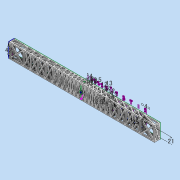
# Autodesk Inventor part: hashi1shado
Saved by Autodesk Inventor 2022 (Build 260153000, 153)
## iProperties
Created: 2024-05-14
Part Number: hashi1shado
Material: 一般
Document SubType Name: Modeling
Designer: ktamu
Density: 1 g/cm^3
Appearance: 既定
Mass: 151.289 g
Surface Area: 1319.93 cm^2
Volume: 151.289 cm^3
Author: ktamu
Autodesk Inventor part; units mm, degrees
ref_plane "YZ Plane" through (0, 0, 0) normal (1, 0, 0) x (0, 1, 0)
ref_plane "XZ Plane" through (0, 0, 0) normal (0, 1, 0) x (-1, 0, 0)
ref_plane "XY Plane" through (0, 0, 0) normal (0, 0, 1) x (1, 0, 0)
sketch "スケッチ2" plane through (0, 0, 0) normal (1, 0, 0) x (0, 1, 0)
  line L0 (25, 10) -> (-25, 10)
  line L1 (-25, 10) -> (-25, -10)
  line L2 (-25, -10) -> (25, -10)
  line L3 (25, -10) -> (25, 10)
  line L4 (25, 10) -> (-25, -10) construction
  line L5 (-25, 10) -> (25, -10) construction
  point P0 (0, 0)
  dimension "d4" = 50
  dimension "d5" = 20
  constraints: 12 end point, 2 midpoint, 2 parallel, 1 horizontal, 1 perpendicular
  measures "d4" distance of L2.end L1.end
  measures "d5" distance of L1.end L0.end
extrude "押し出し2" add sketch "スケッチ2" along normal mid plane 500
sketch "スケッチ3" plane through (-250, -25, 10) normal (0, 0, 1) x (1, 0, 0)
  circle A0 centre (250, 25) radius 5
  dimension "d8" = 10
  constraints: 1 centre point, 1 coincident
  measures "d8" diameter of A0
extrude "押し出し3" add sketch "スケッチ3" along normal blind 2
sketch "SCLeft" plane through (-250, 0, 0) normal (-1, 0, 0) x (0, 0, 1)
  line L0 (10, 25) -> (10, -25) projected
  line L1 (-10, 25) -> (10, 25)
  line L2 (10, 25) -> (10, -25)
  line L3 (10, -25) -> (-10, -25)
  line L4 (-10, -25) -> (-10, 25)
  line L5 (-10, 25) -> (10, -25) construction
  line L6 (10, 25) -> (-10, -25) construction
  line L7 (-6, 21) -> (6, 21)
  line L8 (6, 21) -> (6, -21)
  line L9 (6, -21) -> (-6, -21)
  line L10 (-6, -21) -> (-6, 21)
  line L11 (-6, 21) -> (-1.04, 3.6401) construction
  line L12 (6, 21) -> (-6, -21) construction
  line L13 (7.4154, 0) -> (4.3427, 0)
  line L14 (2.08, 0) -> (6, -13.7199)
  line L15 (-3.92, 21) -> (0, 7.2801)
  line L16 (-6, 21) -> (-1.04, 3.6401)
  line L17 (1.04, -3.6401) -> (6, -21)
  line L18 (-6, 13.7199) -> (-2.08, 0)
  line L19 (0, -7.2801) -> (3.92, -21)
  line L20 (0, 7.2801) -> (3.92, 21)
  line L21 (-6, -13.7199) -> (-2.08, 0)
  line L22 (-3.92, -21) -> (0, -7.2801)
  line L23 (2.08, 0) -> (6, 13.7199)
  point P0 (0, 0)
  dimension "d47" = 12
  dimension "d48" = 42
  constraints: 46 end point, 8 parallel, 5 point on line, 4 symmetric about line, 3 horizontal, 3 midpoint, 2 perpendicular
  measures "d47" distance of L8.end L9.end
  measures "d48" distance of L7.end L8.end
extrude "押し出し5left" cut sketch "SCLeft" against normal through all contours L7 L15 L20 L8 L23 L14 L9 L19 L22 L10 L21 L18 | L7 L20 L15 | L18 L21 L10 | L8 L14 L23 | L22 L19 L9
extrude "押し出し6" add sketch "SCLeft" against normal blind 4 contours L7 L15 L20 L8 L23 L14 L9 L19 L22 L10 L21 L18
mirror "ミラー1" about plane through (0, 0, 0) normal (1, 0, 0) of "押し出し6"
sketch "SCtop" plane through (-250, -25, 10) normal (0, 0, 1) x (1, 0, 0)
  circle A0 centre (250, 25) radius 5 projected
  line L0 (500, 0) -> (0, 0) projected
  line L1 (500, 50) -> (500, 0) projected
  line L2 (0, 50) -> (500, 50) projected
  line L3 (0, 0) -> (0, 50) projected
  circle A1 centre (250, 25) radius 5 projected
  line L4 (0, 0) -> (0, 50) projected
  line L5 (0, 50) -> (500, 0) construction
  line L6 (0, 0) -> (500, 0) projected
  line L7 (500, 50) -> (0, 0) construction
  line L8 (0, 50) -> (500, 50)
  line L9 (500, 50) -> (500, 0)
  line L10 (500, 0) -> (0, 0)
  line L11 (0, 0) -> (0, 50)
  line L12 (0, 50) -> (500, 0) construction
  line L13 (500, 50) -> (0, 0) construction
  line L14 (0, 50) -> (500, 50) projected
  line L15 (0, 50) -> (50, 50)
  line L16 (50, 50) -> (50, 0)
  line L17 (50, 0) -> (0, 0)
  line L18 (0, 0) -> (0, 50)
  line L19 (100, 50) -> (100, 0)
  line L20 (150, 50) -> (150, 0)
  line L21 (200, 50) -> (200, 0)
  line L22 (250, 50) -> (250, 0)
  line L23 (300, 50) -> (300, 0)
  line L24 (350, 50) -> (350, 0)
  line L25 (400, 50) -> (400, 0)
  line L26 (450, 50) -> (450, 0)
  line L27 (50, 50) -> (100, 0)
  line L28 (0, 50) -> (50, 0)
  line L29 (50, 50) -> (0, 0)
  line L30 (98, 4) -> (60.1439, 4) projected
  line L31 (52, 46) -> (98, 46)
  line L32 (98, 46) -> (98, 4)
  line L33 (98, 4) -> (52, 4)
  line L34 (52, 4) -> (52, 46)
  line L35 (4, 46) -> (48, 46)
  line L36 (48, 46) -> (48, 4)
  line L37 (48, 4) -> (4, 4)
  line L38 (4, 4) -> (4, 46)
  line L39 (6.8284, 46) -> (48.0258, 4.8026)
  line L40 (4, 43.1716) -> (43.1716, 4)
  line L41 (25, 25) -> (25, 18.6219)
  line L42 (98, 0) -> (98, 4) projected
  line L43 (53.4759, 44.6524) -> (98, 4)
  line L44 (52, 43.2918) -> (95.0338, 4)
  line L45 (54.9662, 46) -> (98, 6.7082)
  line L46 (98, 43.2918) -> (54.9662, 4)
  line L47 (92.2747, 40.7725) -> (53.4759, 5.3476)
  line L48 (95.0338, 46) -> (52, 6.7082)
  line L49 (50.1449, 5.0145) -> (50, 4.8822)
  line L50 (73.5843, 23.5843) -> (90.9091, 40.9091)
  line L51 (92.2747, 40.7725) -> (73.5169, 23.6459) construction
  line L52 (53.4759, 5.3476) -> (52, 4) construction
  line L53 (52, 46) -> (53.4759, 44.6524) construction
  line L54 (73.5169, 26.3541) -> (98, 4) construction
  line L55 (48, 46) -> (4, 4)
  line L56 (45.1034, 46) -> (4, 6.7649)
  line L57 (48, 43.2351) -> (6.8966, 4)
  line L58 (104.9662, 46) -> (148, 6.7082)
  line L59 (145.0338, 46) -> (102, 6.7082)
  line L60 (148, 43.2918) -> (104.9662, 4)
  line L61 (102, 43.2918) -> (145.0338, 4)
  line L62 (148, 46) -> (148, 4)
  line L63 (102, 46) -> (148, 46)
  line L64 (102, 4) -> (102, 46)
  line L65 (148, 4) -> (102, 4)
  line L66 (154.9662, 46) -> (198, 6.7082)
  line L67 (195.0338, 46) -> (152, 6.7082)
  line L68 (198, 43.2918) -> (154.9662, 4)
  line L69 (152, 43.2918) -> (195.0338, 4)
  line L70 (198, 46) -> (198, 4)
  line L71 (152, 46) -> (198, 46)
  line L72 (152, 4) -> (152, 46)
  line L73 (198, 4) -> (152, 4)
  line L74 (204.9662, 46) -> (248, 6.7082)
  line L75 (245.0338, 46) -> (202, 6.7082)
  line L76 (248, 43.2918) -> (204.9662, 4)
  line L77 (202, 43.2918) -> (245.0338, 4)
  line L78 (248, 46) -> (248, 4)
  line L79 (202, 46) -> (248, 46)
  line L80 (202, 4) -> (202, 46)
  line L81 (248, 4) -> (202, 4)
  line L82 (254.9662, 46) -> (298, 6.7082)
  line L83 (295.0338, 46) -> (252, 6.7082)
  line L84 (298, 43.2918) -> (254.9662, 4)
  line L85 (252, 43.2918) -> (295.0338, 4)
  line L86 (298, 46) -> (298, 4)
  line L87 (252, 46) -> (298, 46)
  line L88 (252, 4) -> (252, 46)
  line L89 (298, 4) -> (252, 4)
  line L90 (304.9662, 46) -> (348, 6.7082)
  line L91 (345.0338, 46) -> (302, 6.7082)
  line L92 (348, 43.2918) -> (304.9662, 4)
  line L93 (302, 43.2918) -> (345.0338, 4)
  line L94 (348, 46) -> (348, 4)
  line L95 (302, 46) -> (348, 46)
  line L96 (302, 4) -> (302, 46)
  line L97 (348, 4) -> (302, 4)
  line L98 (354.9662, 46) -> (398, 6.7082)
  line L99 (395.0338, 46) -> (352, 6.7082)
  line L100 (398, 43.2918) -> (354.9662, 4)
  line L101 (352, 43.2918) -> (395.0338, 4)
  line L102 (398, 46) -> (398, 4)
  line L103 (352, 46) -> (398, 46)
  line L104 (352, 4) -> (352, 46)
  line L105 (398, 4) -> (352, 4)
  line L106 (404.9662, 46) -> (448, 6.7082)
  line L107 (445.0338, 46) -> (402, 6.7082)
  line L108 (448, 43.2918) -> (404.9662, 4)
  line L109 (402, 43.2918) -> (445.0338, 4)
  line L110 (448, 46) -> (448, 4)
  line L111 (402, 46) -> (448, 46)
  line L112 (402, 4) -> (402, 46)
  line L113 (448, 4) -> (402, 4)
  line L114 (496, 46) -> (452, 46)
  line L115 (452, 46) -> (452, 4)
  line L116 (452, 4) -> (496, 4)
  line L117 (496, 4) -> (496, 46)
  line L118 (493.1716, 46) -> (451.9742, 4.8026)
  line L119 (496, 43.1716) -> (456.8284, 4)
  line L120 (454.8966, 46) -> (496, 6.7649)
  line L121 (452, 43.2351) -> (493.1034, 4)
  point P0 (75, 25)
  point P1 (123.5169, 26.3541)
  point P2 (123.5843, 23.5843)
  point P3 (123.5169, 23.6459)
  point P4 (173.5169, 26.3541)
  point P5 (173.5843, 23.5843)
  point P6 (173.5169, 23.6459)
  point P7 (223.5169, 26.3541)
  point P8 (223.5843, 23.5843)
  point P9 (223.5169, 23.6459)
  point P10 (273.5169, 26.3541)
  point P11 (273.5843, 23.5843)
  point P12 (273.5169, 23.6459)
  point P13 (323.5169, 26.3541)
  point P14 (323.5843, 23.5843)
  point P15 (323.5169, 23.6459)
  point P16 (373.5169, 26.3541)
  point P17 (373.5843, 23.5843)
  point P18 (373.5169, 23.6459)
  point P19 (423.5169, 26.3541)
  point P20 (423.5843, 23.5843)
  point P21 (423.5169, 23.6459)
  point P22 (474.5441, 21.7157)
  point P23 (477.3733, 24.5449)
  point P24 (474.4791, 27.3075)
  point P25 (452, 4.8284)
  point P26 (471.6499, 24.4784)
  point P27 (427.9662, 25)
  point P28 (425, 22.2918)
  point P29 (425, 27.7082)
  point P30 (375, 22.2918)
  point P31 (375, 27.7082)
  point P32 (422.0338, 25)
  point P33 (377.9662, 25)
  point P34 (372.0338, 25)
  point P35 (327.9662, 25)
  point P36 (325, 22.2918)
  point P37 (325, 27.7082)
  point P38 (322.0338, 25)
  point P39 (275, 22.2918)
  point P40 (277.9662, 25)
  point P41 (275, 27.7082)
  point P42 (252, 20.4174)
  point P43 (272.0338, 25)
  point P44 (252, 29.5826)
  point P45 (225, 22.2918)
  point P46 (248, 29.5826)
  point P47 (227.9662, 25)
  point P48 (248, 20.4174)
  point P49 (225, 27.7082)
  point P50 (222.0338, 25)
  point P51 (175, 22.2918)
  point P52 (177.9662, 25)
  point P53 (175, 27.7082)
  point P54 (172.0338, 25)
  point P55 (125, 22.2918)
  point P56 (127.9662, 25)
  point P57 (125, 27.7082)
  point P58 (122.0338, 25)
  point P59 (77.9662, 25)
  point P60 (75, 22.2918)
  point P61 (75, 27.7082)
  point P62 (72.0338, 25)
  point P63 (25.4559, 21.7157)
  point P64 (28.3501, 24.4784)
  point P65 (48, 4.8284)
  point P66 (22.6267, 24.5449)
  point P67 (25.5209, 27.3075)
  dimension "d55" = 50
  dimension "d56" = 50
  dimension "d59" = 50
  dimension "d64" = 46
  dimension "d65" = 42
  dimension "d66" = 44
  dimension "d67" = 42
  dimension "d68" = 4
  dimension "d69" = 4
  dimension "d76" = 2
  dimension "d77" = 2
  dimension "d80" = 50
  constraints: 226 end point, 97 point on line, 20 midpoint, 17 parallel, 12 symmetric about line, 6 horizontal, 5 perpendicular, 1 vertical, 185 other
  measures "d55" distance of L16.end L17.end
  measures "d56" distance of L15.end L16.end
  measures "d59" distance of L15.end L19.start
  measures "d64" distance of L30.start L33.end
  measures "d65" distance of L31.end L30.start
  measures "d66" distance of L36.end L37.end
  measures "d67" distance of L35.end L36.end
  measures "d68" distance between parallel lines of L2 L35
  measures "d69" distance between parallel lines of L34 L36
  measures "d76" distance between parallel lines of L55 L56
  measures "d77" distance between parallel lines of L55 L57
  measures "d80" distance of L45.start L58.start
sketch "スケッチ7" plane through (0, 0, 12) normal (0, 0, 1) x (1, 0, 0)
  line L0 (-2, 21) -> (-2, -21) projected
  line L1 (2, -18.2918) -> (2, 0) projected
  line L2 (2, -21) -> (2, 21) projected
  circle A0 centre (0, 0) radius 5 projected
  arc A1 (5, 0) -> (5, 0) centre (0, 0) ccw projected
  line L3 (5, 0) -> (-2, 4.5826)
  line L4 (5, 0) -> (2, 4.5826)
  circle A2 centre (0, 0) radius 1
  point P0 (-2, -21)
  point P1 (2, 21)
  point P2 (2, -4.5826)
  point P3 (-2, -4.5826)
  dimension "d89" = 2
  constraints: 4 end point, 2 point on circle, 1 centre point, 1 coincident, 4 other
  measures "d89" diameter of A2
extrude "押し出し8" cut sketch "スケッチ7" against normal through all contours L0 A0 | L4 L3 L2 | A0 L4 | L3 A0 L1 L2
extrude "押し出し9" cut sketch "スケッチ7" against normal blind 2 contours L3 L2 L1 A0 L0 | A0 L2 L3
extrude "押し出し10" cut sketch "スケッチ7" against normal blind 1 contours A2
sketch "スケッチ8" plane through (-250, 25, 10) normal (0, 1, 0) x (1, 0, 0)
  point P0 (250, 10)
sketch "スケッチ10" plane through (-250, 25, 10) normal (0, 1, 0) x (1, 0, 0)
  point P0 (250, 10)
sketch "SCfronNNhukin" plane through (-250, -25, -10) normal (0, -1, 0) x (1, 0, 0)
  line L0 (0, -20) -> (500, -20)
  line L1 (500, 0) -> (500, -20)
  line L2 (500, 0) -> (0, 0)
  line L3 (0, -20) -> (0, 0)
  line L4 (0, 0) -> (500, 0)
  line L5 (500, 0) -> (500, -20)
  line L6 (500, -20) -> (0, -20)
  line L7 (0, -20) -> (0, 0)
  line L8 (0, 0) -> (500, -20) construction
  line L9 (500, 0) -> (0, -20) construction
  line L10 (0, 0) -> (500, 0)
  line L11 (0, -20) -> (500, -20)
  line L12 (0, 0) -> (50, 0)
  line L13 (50, 0) -> (50, -20)
  line L14 (50, -20) -> (0, -20)
  line L15 (0, -20) -> (0, 0)
  line L16 (100, 0) -> (100, -20)
  line L17 (150, 0) -> (150, -20)
  line L18 (200, 0) -> (200, -20)
  line L19 (250, 0) -> (250, -20)
  line L20 (450, 0) -> (450, -20)
  line L21 (400, 0) -> (400, -20)
  line L22 (350, 0) -> (350, -20)
  line L23 (300, 0) -> (300, -20)
  line L24 (0, 0) -> (0, -20)
  line L25 (0, 0) -> (50, -20)
  line L26 (0, -20) -> (50, 0) construction
  line L27 (50, 0) -> (100, -20)
  line L28 (100, 0) -> (50, -20)
  line L29 (52, -4) -> (98, -4)
  line L30 (98, -4) -> (98, -16)
  line L31 (98, -16) -> (52, -16)
  line L32 (52, -16) -> (52, -4)
  line L33 (75, -10) -> (98, -16) construction
  line L34 (98, -4) -> (52, -16) construction
  line L35 (102, -4) -> (148, -4)
  line L36 (102, -16) -> (102, -4)
  line L37 (148, -16) -> (102, -16)
  line L38 (148, -4) -> (148, -16)
  line L39 (152, -4) -> (198, -4)
  line L40 (152, -16) -> (152, -4)
  line L41 (198, -16) -> (152, -16)
  line L42 (198, -4) -> (198, -16)
  line L43 (202, -4) -> (248, -4)
  line L44 (202, -16) -> (202, -4)
  line L45 (248, -16) -> (202, -16)
  line L46 (248, -4) -> (248, -16)
  line L47 (252, -4) -> (298, -4)
  line L48 (252, -16) -> (252, -4)
  line L49 (298, -16) -> (252, -16)
  line L50 (298, -4) -> (298, -16)
  line L51 (302, -4) -> (348, -4)
  line L52 (302, -16) -> (302, -4)
  line L53 (348, -16) -> (302, -16)
  line L54 (348, -4) -> (348, -16)
  line L55 (352, -4) -> (398, -4)
  line L56 (352, -16) -> (352, -4)
  line L57 (398, -16) -> (352, -16)
  line L58 (398, -4) -> (398, -16)
  line L59 (402, -4) -> (448, -4)
  line L60 (402, -16) -> (402, -4)
  line L61 (448, -16) -> (402, -16)
  line L62 (448, -4) -> (448, -16)
  line L63 (48, -4) -> (48, -16)
  line L64 (48, -4) -> (4, -4)
  line L65 (4, -4) -> (4, -16)
  line L66 (4, -16) -> (48, -16)
  line L67 (48, -16) -> (48, -4)
  line L68 (452, -4) -> (496, -4)
  line L69 (496, -4) -> (496, -16)
  line L70 (496, -16) -> (452, -16)
  line L71 (452, -4) -> (452, -16)
  line L72 (11.4052, -4) -> (48, -14.2649)
  line L73 (4, -6.0772) -> (40.5948, -16)
  line L74 (488.5948, -4) -> (452, -14.2649)
  line L75 (496, -6.0772) -> (459.4052, -16)
  line L76 (52, -4) -> (75, -10)
  line L77 (52, -6.0669) -> (90.0768, -16)
  line L78 (52.5048, -2.0648) -> (52.6652, -2.1066)
  line L79 (59.9232, -4) -> (98, -13.9331)
  line L80 (109.9232, -4) -> (148, -13.9331)
  line L81 (102, -6.0669) -> (140.0768, -16)
  line L82 (159.9232, -4) -> (198, -13.9331)
  line L83 (152, -6.0669) -> (190.0768, -16)
  line L84 (209.9232, -4) -> (248, -13.9331)
  line L85 (202, -6.0669) -> (240.0768, -16)
  line L86 (448, -6.0669) -> (409.9232, -16)
  line L87 (440.0768, -4) -> (402, -13.9331)
  line L88 (398, -6.0669) -> (359.9232, -16)
  line L89 (390.0768, -4) -> (352, -13.9331)
  line L90 (348, -6.0669) -> (309.9232, -16)
  line L91 (340.0768, -4) -> (302, -13.9331)
  line L92 (298, -6.0669) -> (259.9232, -16)
  line L93 (290.0768, -4) -> (252, -13.9331)
  line L94 (500, 20) -> (0, 20)
  line L95 (0, 20) -> (500, 20)
  line L96 (0, 20) -> (500, 20)
  line L97 (0, 0) -> (500, 0)
  line L98 (500, 0) -> (0, 0)
  line L99 (0, 0) -> (500, 0)
  line L100 (0, 20) -> (500, 0) construction
  line L101 (500, 20) -> (0, 0) construction
  line L102 (352, 4) -> (352, 16)
  line L103 (352, 16) -> (398, 16)
  line L104 (398, 4) -> (352, 4)
  line L105 (398, 13.9331) -> (359.9232, 4)
  line L106 (398, 16) -> (398, 4)
  line L107 (390.0768, 16) -> (352, 6.0669)
  line L108 (440.0768, 16) -> (402, 6.0669)
  line L109 (448, 16) -> (448, 4)
  line L110 (448, 13.9331) -> (409.9232, 4)
  line L111 (448, 4) -> (402, 4)
  line L112 (402, 16) -> (448, 16)
  line L113 (400, 20) -> (400, 0)
  line L114 (202, 4) -> (202, 16)
  line L115 (202, 13.9331) -> (240.0768, 4)
  line L116 (202, 16) -> (248, 16)
  line L117 (248, 4) -> (202, 4)
  line L118 (209.9232, 16) -> (248, 6.0669)
  line L119 (248, 16) -> (248, 4)
  line L120 (148, 16) -> (148, 4)
  line L121 (109.9232, 16) -> (148, 6.0669)
  line L122 (102, 16) -> (148, 16)
  line L123 (102, 4) -> (102, 16)
  line L124 (102, 13.9331) -> (140.0768, 4)
  line L125 (148, 4) -> (102, 4)
  line L126 (300, 20) -> (300, 0)
  line L127 (302, 4) -> (302, 16)
  line L128 (340.0768, 16) -> (302, 6.0669)
  line L129 (348, 4) -> (302, 4)
  line L130 (302, 16) -> (348, 16)
  line L131 (348, 13.9331) -> (309.9232, 4)
  line L132 (348, 16) -> (348, 4)
  line L133 (350, 20) -> (350, 0)
  line L134 (402, 4) -> (402, 16)
  line L135 (75, 10) -> (98, 4) construction
  line L136 (98, 16) -> (98, 4)
  line L137 (100, 20) -> (100, 0)
  line L138 (59.9232, 16) -> (98, 6.0669)
  line L139 (52.5048, 17.9352) -> (52.6652, 17.8934)
  line L140 (52, 13.9331) -> (90.0768, 4)
  line L141 (52, 4) -> (52, 16)
  line L142 (52, 16) -> (75, 10)
  line L143 (50, 20) -> (50, 0)
  line L144 (52, 16) -> (98, 16)
  line L145 (50, 20) -> (100, 0)
  line L146 (100, 20) -> (50, 0)
  line L147 (98, 16) -> (52, 4) construction
  line L148 (98, 4) -> (52, 4)
  line L149 (0, 0) -> (0, 20)
  line L150 (0, 0) -> (0, 20)
  line L151 (48, 16) -> (48, 4)
  line L152 (48, 4) -> (48, 16)
  line L153 (11.4052, 16) -> (48, 5.7351)
  line L154 (4, 4) -> (48, 4)
  line L155 (4, 13.9228) -> (40.5948, 4)
  line L156 (4, 16) -> (4, 4)
  line L157 (50, 0) -> (0, 0)
  line L158 (0, 20) -> (50, 0)
  line L159 (0, 0) -> (50, 20) construction
  line L160 (0, 20) -> (50, 20)
  line L161 (48, 16) -> (4, 16)
  line L162 (0, 20) -> (0, 0)
  line L163 (0, 0) -> (0, 20)
  line L164 (500, 20) -> (500, 0)
  line L165 (500, 20) -> (500, 0)
  line L166 (450, 20) -> (450, 0)
  line L167 (452, 16) -> (452, 4)
  line L168 (488.5948, 16) -> (452, 5.7351)
  line L169 (452, 16) -> (496, 16)
  line L170 (496, 4) -> (452, 4)
  line L171 (496, 16) -> (496, 4)
  line L172 (496, 13.9228) -> (459.4052, 4)
  line L173 (200, 20) -> (200, 0)
  line L174 (198, 16) -> (198, 4)
  line L175 (159.9232, 16) -> (198, 6.0669)
  line L176 (198, 4) -> (152, 4)
  line L177 (152, 13.9331) -> (190.0768, 4)
  line L178 (152, 4) -> (152, 16)
  line L179 (150, 20) -> (150, 0)
  line L180 (152, 16) -> (198, 16)
  line L181 (250, 20) -> (250, 0)
  line L182 (298, 16) -> (298, 4)
  line L183 (298, 13.9331) -> (259.9232, 4)
  line L184 (252, 16) -> (298, 16)
  line L185 (298, 4) -> (252, 4)
  line L186 (290.0768, 16) -> (252, 6.0669)
  line L187 (252, 4) -> (252, 16)
  line L188 (0, 0) -> (500, 0) projected
  line L189 (500, 20) -> (500, 0) projected
  line L190 (500, 20) -> (0, 20) projected
  line L191 (0, 0) -> (0, 20) projected
  line L192 (75, 10) -> (75, 16) construction
  line L193 (75, 10) -> (75, 4) construction
  line L194 (73, 10) -> (73, 16)
  line L195 (73, 10) -> (73, 4)
  line L196 (77, 10) -> (77, 16)
  line L197 (77, 10) -> (77, 4)
  line L198 (52, 16) -> (73, 16)
  line L199 (73, 16) -> (73, 4)
  line L200 (73, 4) -> (52, 4)
  line L201 (52, 4) -> (52, 16)
  line L202 (77, 16) -> (98, 16)
  line L203 (98, 16) -> (98, 4)
  line L204 (98, 4) -> (77, 4)
  line L205 (77, 4) -> (77, 16)
  line L206 (52, 16) -> (73, 4)
  line L207 (73, 16) -> (52, 4)
  line L208 (86.0655, 9.1803) -> (77, 4)
  line L209 (56.0311, 16) -> (73, 6.3035)
  line L210 (98, 13.6965) -> (81.0311, 4)
  line L211 (80.9911, 16) -> (98.4974, 5.8625)
  line L212 (77, 13.6889) -> (96.4929, 2.4009)
  line L213 (89.4323, 8.8007) -> (97.4952, 4.1317)
  line L214 (82.3111, 12.9244) -> (83.5221, 12.2232)
  line L215 (85.428, 11.1195) -> (87.4302, 9.9601)
  line L216 (94.3634, 16.2255) -> (85.428, 11.1195)
  line L217 (83.4192, 9.9716) -> (77, 6.3035)
  line L218 (52, 13.6965) -> (68.9689, 4)
  line L219 (69.0089, 16) -> (52, 6.1505)
  line L220 (73, 13.6889) -> (56.2685, 4)
  line L221 (56.0311, 16) -> (64.572, 11.1195)
  line L222 (66.5808, 9.9716) -> (73, 6.3035)
  line L223 (52, 13.6965) -> (68.9689, 4)
  line L224 (102, 13.6965) -> (118.9689, 4)
  line L225 (106.0311, 16) -> (123, 6.3035)
  line L226 (119.0089, 16) -> (102, 6.1505)
  line L227 (123, 13.6889) -> (106.2685, 4)
  line L228 (130.9911, 16) -> (148.4974, 5.8625)
  line L229 (127, 13.6889) -> (146.4929, 2.4009)
  line L230 (133.4192, 9.9716) -> (127, 6.3035)
  line L231 (144.3634, 16.2255) -> (135.428, 11.1195)
  line L232 (148, 13.6965) -> (131.0311, 4)
  line L233 (148, 4) -> (102, 4)
  line L234 (123, 10) -> (123, 4)
  line L235 (123, 10) -> (123, 16)
  line L236 (102, 16) -> (148, 16)
  line L237 (102, 4) -> (102, 16)
  line L238 (102, 16) -> (123, 16)
  line L239 (102, 4) -> (102, 16)
  line L240 (123, 4) -> (102, 4)
  line L241 (127, 4) -> (127, 16)
  line L242 (148, 4) -> (127, 4)
  line L243 (148, 16) -> (148, 4)
  line L244 (127, 16) -> (148, 16)
  line L245 (4, 16) -> (4, 13.92) projected
  line L246 (4, 16) -> (48, 16)
  line L247 (48, 16) -> (48, 4)
  line L248 (48, 4) -> (4, 4)
  line L249 (4, 4) -> (4, 16)
  line L250 (198, 4) -> (186, 4)
  line L251 (186, 4) -> (186, 16)
  line L252 (186, 16) -> (198, 16)
  line L253 (198, 16) -> (198, 4)
  line L254 (152, 16) -> (165, 16)
  line L255 (165, 16) -> (165, 4)
  line L256 (165, 4) -> (152, 4)
  line L257 (152, 4) -> (152, 16)
  line L258 (4, 16) -> (496, 16) projected
  line L259 (169, 16) -> (182, 16)
  line L260 (182, 16) -> (182, 4)
  line L261 (182, 4) -> (169, 4)
  line L262 (169, 4) -> (169, 16)
  line L263 (152, 16) -> (165, 4) construction
  line L264 (169, 16) -> (182, 4)
  line L265 (150, 18) -> (149.8333, 18)
  line L266 (167, 13.32) -> (167, 16)
  line L267 (166.0425, 2.094) -> (168.2361, 1.5218)
  line L268 (167, 1.8442) -> (167, 6.68)
  line L269 (154.9486, 16) -> (165.1265, 6.6051)
  line L270 (167, 4.8757) -> (169.7131, 2.3712)
  line L271 (152, 13.2782) -> (162.0514, 4)
  line L272 (166.3847, 0) -> (167, -0.568)
  line L273 (184, 18) -> (169, 18)
  line L274 (167, 18) -> (166.8333, 18)
  line L275 (184, 4) -> (184, 18)
  line L276 (171.9486, 16) -> (182, 6.7218)
  line L277 (163.8847, 18) -> (167, 15.1243)
  line L278 (168.4655, 13.7716) -> (179.0514, 4)
  line L279 (183.3847, 0) -> (184, -0.568)
  line L280 (169, 4) -> (182, 4)
  line L281 (186, 4) -> (198, 4)
  line L282 (186, 16) -> (198, 4)
  line L283 (184, 18) -> (184, 4)
  line L284 (186, 13.1716) -> (195.1716, 4)
  line L285 (186, 16) -> (198, 4)
  line L286 (188.8284, 16) -> (198, 6.8284)
  line L287 (248, 16) -> (239.5, 16)
  line L288 (239.5, 16) -> (239.5, 4)
  line L289 (239.5, 4) -> (248, 4)
  line L290 (248, 4) -> (248, 16)
  line L291 (235.5, 16) -> (227, 16)
  line L292 (227, 16) -> (227, 4)
  line L293 (227, 4) -> (235.5, 4)
  line L294 (235.5, 4) -> (235.5, 16)
  line L295 (225, 20) -> (225, 22.2836)
  line L296 (229.4509, 16) -> (235.5, 7.4601)
  line L297 (227, 12.5399) -> (233.0491, 4)
  line L298 (230.7033, 10.7719) -> (230.8707, 10.5354)
  line L299 (234.4626, 5.4646) -> (235.5, 4)
  line L300 (239.5, 12.5399) -> (245.5491, 4)
  line L301 (241.9509, 16) -> (248, 7.4601)
  line L302 (214.5, 16) -> (214.5, 4)
  line L303 (223, 16) -> (214.5, 16)
  line L304 (216.9509, 16) -> (223, 7.4601)
  line L305 (223, 4) -> (223, 16)
  line L306 (214.5, 4) -> (223, 4)
  line L307 (214.5, 12.5399) -> (220.5491, 4)
  line L308 (202, 16) -> (202, 4)
  line L309 (210.5, 16) -> (202, 16)
  line L310 (204.4509, 16) -> (210.5, 7.4601)
  line L311 (210.5, 4) -> (210.5, 16)
  line L312 (202, 4) -> (210.5, 4)
  line L313 (202, 12.5399) -> (208.0491, 4)
  line L314 (11.4052, 16) -> (48, 5.7351)
  line L315 (4, 13.9228) -> (40.5948, 4)
  point P0 (250, 10)
  point P1 (250, -10)
  point P2 (250, 10)
  point P3 (55.6366, 16.2255)
  point P4 (51.5026, 5.8625)
  point P5 (53.5071, 2.4009)
  point P6 (116.5808, 9.9716)
  point P7 (139.4323, 8.8007)
  point P8 (125, 4)
  point P9 (125, 16)
  point P10 (127, 4)
  point P11 (189.0701, 9.6559)
  point P12 (195.1716, 4)
  point P13 (169, 13.2782)
  point P14 (165, 6.7218)
  point P15 (148, 6.1505)
  point P16 (141.4411, 9.9486)
  point P17 (143.9689, 16)
  point P18 (137.4368, 12.2674)
  point P19 (143.7315, 4)
  point P20 (77, 13.6889)
  point P21 (77, 10)
  point P22 (77, 4)
  point P23 (93.7315, 4)
  point P24 (98, 6.1505)
  point P25 (68.9689, 4)
  point P26 (4, 13.9228)
  point P27 (11.4052, 16)
  point P28 (48, 5.7351)
  dimension "d106" = 50
  dimension "d107" = 50
  dimension "d108" = 46
  dimension "d109" = 12
  dimension "d110" = 50
  dimension "d111" = 4
  dimension "d112" = 4
  dimension "d113" = 4
  dimension "d114" = 2
  dimension "d115" = 50
  dimension "d121" = 20
  dimension "d126" = 2
  dimension "d127" = 2
  dimension "d128" = 2
  dimension "d129" = 2
  dimension "d131" = 2
  dimension "d133" = 2
  dimension "d138" = 50
  dimension "d143" = 4
  dimension "d144" = 12
  dimension "d145" = 12
  dimension "d146" = 13
  dimension "d147" = 12
  dimension "d148" = 4
  dimension "d149" = 4
  dimension "d155" = 4
  dimension "d156" = 2
  dimension "d157" = 4
  dimension "d158" = 8.5
  dimension "d159" = 12
  dimension "d160" = 8.5
  dimension "d161" = 12
  dimension "d162" = 4
  dimension "d165" = 4
  dimension "d168" = 12.5
  dimension "d175" = 12.5
  dimension "d194" = 20
  constraints: 620 end point, 95 point on line, 64 parallel, 43 symmetric about line, 20 horizontal alignment, 16 horizontal, 16 perpendicular, 11 midpoint, 7 collinear, 3 vertical, 364 other
  measures "d106" distance of L13.end L14.end
  measures "d107" distance of L13.start L16.start
  measures "d108" distance of L31.start L32.start
  measures "d109" distance of L29.end L31.start
  measures "d110" distance of L32.end L35.start
  measures "d111" distance between parallel lines of L32 L63
  measures "d112" distance between parallel lines of L65 L3
  measures "d113" distance between parallel lines of L12 L64
  measures "d114" distance between parallel lines of L76 L77
  measures "d115" distance of L79.start L80.start
  measures "d121" distance of L2.start L94.start
  measures "d126" distance between parallel lines of L192 L194
  measures "d127" distance between parallel lines of L193 L195
  measures "d128" distance between parallel lines of L192 L196
  measures "d129" distance between parallel lines of L193 L197
  measures "d131" distance between parallel lines of L206 L209
  measures "d133" distance between parallel lines of L208 L210
  measures "d138" distance of L218.start L224.start
  measures "d143" distance between parallel lines of L2 L248
  measures "d144" distance of L251.end L252.end
  measures "d145" distance of L250.end L251.end
  measures "d146" distance of L255.end L256.end
  measures "d147" distance of L254.end L255.end
  measures "d148" distance between parallel lines of L262 L255
  measures "d149" distance between parallel lines of L251 L260
  measures "d155" distance between parallel lines of L276 L278
  measures "d156" distance between parallel lines of L284 L285
  measures "d157" distance between parallel lines of L286 L284
  measures "d158" distance of L289.end L288.end
  measures "d159" distance of L288.end L287.end
  measures "d160" distance of L293.end L292.end
  measures "d161" distance of L292.end L291.end
  measures "d162" distance between parallel lines of L288 L294
  measures "d165" distance between parallel lines of L296 L297
  measures "d168" distance of L297.start L300.start
  measures "d175" distance of L291.end L302.start
  measures "d194" distance of L72.start L314.start
sketch "SCBottom" plane through (250, 25, -10) normal (0, 0, -1) x (-1, 0, 0)
  line L0 (77, 10) -> (77, 16)
  line L1 (77, 10) -> (77, 4)
  line L2 (73, 16) -> (73, 4)
  line L3 (52, 4) -> (52, 16)
  line L4 (98, 16) -> (98, 4)
  line L5 (123, 10) -> (123, 4)
  line L6 (123, 10) -> (123, 16)
  line L7 (102, 4) -> (102, 16)
  line L8 (127, 4) -> (127, 16)
  line L9 (148, 16) -> (148, 4)
  line L10 (48, 16) -> (48, -57.3207)
  line L11 (186, 4) -> (186, 16)
  line L12 (198, 16) -> (198, 4)
  line L13 (165, 16) -> (165, 4)
  line L14 (152, 4) -> (152, 16)
  line L15 (182, 16) -> (182, 4)
  line L16 (169, 4) -> (169, 16)
  line L17 (239.5, 16) -> (239.5, 4)
  line L18 (248, 4) -> (248, 16)
  line L19 (227, 16) -> (227, 4)
  line L20 (235.5, 4) -> (235.5, 16)
  line L21 (214.5, 16) -> (214.5, 4)
  line L22 (223, 4) -> (223, 16)
  line L23 (202, 16) -> (202, 4)
  line L24 (210.5, 4) -> (210.5, 16)
  arc A0 (248, -20.4174) -> (248, -29.5826) centre (250, -25) ccw projected
  line L25 (248, -20.4174) -> (248, -29.5826) projected
  arc A1 (252, -29.5826) -> (252, -20.4174) centre (250, -25) ccw projected
  line L26 (252, -29.5826) -> (252, -20.4174) projected
  line L27 (500, 0) -> (0, 0) projected
  line L28 (0, -50) -> (0, 0) projected
  line L29 (500, -50) -> (0, -50) projected
  line L30 (500, 0) -> (500, -50) projected
  line L31 (169, -26) -> (169, -14)
  line L32 (165, -14) -> (165, -26)
  line L33 (152, -26) -> (152, -14)
  line L34 (148, -14) -> (148, -26)
  line L35 (127, -26) -> (127, -14)
  line L36 (123, -20) -> (123, -26)
  line L37 (123, -20) -> (123, -14)
  line L38 (102, -26) -> (102, -14)
  line L39 (98, -14) -> (98, -26)
  line L40 (77, -20) -> (77, -14)
  line L41 (77, -20) -> (77, -26)
  line L42 (73, -14) -> (73, -26)
  line L43 (52, -26) -> (52, -14)
  line L44 (496, -4) -> (4, -4) projected
  line L45 (496, -46) -> (4, -46) projected
  line L46 (52, -4) -> (73, -4)
  line L47 (73, -4) -> (73, -46)
  line L48 (73, -46) -> (52, -46)
  line L49 (52, -46) -> (52, -4)
  line L50 (77, -4) -> (98, -4)
  line L51 (98, -4) -> (98, -46)
  line L52 (98, -46) -> (77, -46)
  line L53 (77, -46) -> (77, -4)
  line L54 (102, -4) -> (123, -4)
  line L55 (123, -4) -> (123, -46)
  line L56 (123, -46) -> (102, -46)
  line L57 (102, -46) -> (102, -4)
  line L58 (127, -4) -> (148, -4)
  line L59 (148, -4) -> (148, -46)
  line L60 (148, -46) -> (127, -46)
  line L61 (127, -46) -> (127, -4)
  line L62 (152, -4) -> (165, -4)
  line L63 (165, -4) -> (165, -46)
  line L64 (165, -46) -> (152, -46)
  line L65 (152, -46) -> (152, -4)
  line L66 (169, -4) -> (182, -4)
  line L67 (182, -4) -> (182, -46)
  line L68 (182, -46) -> (169, -46)
  line L69 (169, -46) -> (169, -4)
  line L70 (186, -4) -> (198, -4)
  line L71 (198, -4) -> (198, -46)
  line L72 (198, -46) -> (186, -46)
  line L73 (186, -46) -> (186, -4)
  line L74 (210.5, -4) -> (214.5, -4)
  line L75 (214.5, -4) -> (214.5, -46)
  line L76 (214.5, -46) -> (210.5, -46)
  line L77 (210.5, -46) -> (210.5, -4)
  line L78 (223, -4) -> (227, -4)
  line L79 (227, -4) -> (227, -46)
  line L80 (227, -46) -> (223, -46)
  line L81 (223, -46) -> (223, -4)
  line L82 (235.5, -4) -> (239.5, -4)
  line L83 (239.5, -4) -> (239.5, -46)
  line L84 (239.5, -46) -> (235.5, -46)
  line L85 (235.5, -46) -> (235.5, -4)
  line L86 (248, -4) -> (252, -4)
  line L87 (252, -4) -> (252, -46)
  line L88 (252, -46) -> (248, -46)
  line L89 (248, -46) -> (248, -4)
  line L90 (52, -25) -> (252, -25)
  line L91 (62.5, -25) -> (52, -4)
  line L92 (88.618, -27.2361) -> (77, -4)
  line L93 (123, -46) -> (102, -4)
  line L94 (127, -4) -> (148, -46)
  line L95 (182, -46) -> (169, -4)
  line L96 (192, -25) -> (198, -46)
  line L97 (202, -4) -> (202, -46)
  line L98 (223, -46) -> (214.5, -4)
  line L99 (70.7639, -46) -> (52, -8.4721)
  line L100 (73, -41.5279) -> (54.2361, -4)
  line L101 (70.7639, -4) -> (52, -41.5279)
  line L102 (73, -8.4721) -> (54.2361, -46)
  line L103 (98, -41.5279) -> (79.2361, -4)
  line L104 (95.7639, -46) -> (77, -8.4721)
  line L105 (98, -8.4721) -> (79.2361, -46)
  line L106 (95.7639, -4) -> (77, -41.5279)
  line L107 (98, -41.5279) -> (79.2361, -4)
  line L108 (95.7639, -46) -> (77, -8.4721)
  line L109 (98, -8.4721) -> (79.2361, -46)
  line L110 (95.7639, -4) -> (77, -41.5279)
  line L111 (123, -41.5279) -> (104.2361, -4)
  line L112 (120.7639, -46) -> (102, -8.4721)
  line L113 (123, -8.4721) -> (104.2361, -46)
  line L114 (120.7639, -4) -> (102, -41.5279)
  line L115 (148, -41.5279) -> (129.2361, -4)
  line L116 (145.7639, -46) -> (127, -8.4721)
  line L117 (148, -8.4721) -> (129.2361, -46)
  line L118 (145.7639, -4) -> (127, -41.5279)
  line L119 (162.9064, -46) -> (152, -10.764)
  line L120 (165, -39.236) -> (154.0936, -4)
  line L121 (165, -10.764) -> (160.5936, -25)
  line L122 (158.5, -31.764) -> (154.0936, -46)
  line L123 (162.9064, -4) -> (158.5, -18.236)
  line L124 (156.4064, -25) -> (152, -39.236)
  line L125 (157.4532, -21.618) -> (152, -4)
  line L126 (179.9064, -46) -> (169, -10.764)
  line L127 (175.5, -31.764) -> (171.0936, -46)
  line L128 (173.4064, -25) -> (169, -39.236)
  line L129 (182, -39.236) -> (171.0936, -4)
  line L130 (182, -10.764) -> (177.5936, -25)
  line L131 (179.9064, -4) -> (175.5, -18.236)
  line L132 (186, -11.2801) -> (195.92, -46)
  line L133 (188.08, -4) -> (198, -38.7199)
  line L134 (186, -38.7199) -> (195.92, -4)
  line L135 (188.08, -46) -> (198, -11.2801)
  line L136 (235.5, -46) -> (227, -46)
  line L137 (227, -46) -> (227, -4)
  line L138 (227, -4) -> (235.5, -4)
  line L139 (235.5, -4) -> (235.5, -46)
  line L140 (223, -46) -> (214.5, -46)
  line L141 (214.5, -46) -> (214.5, -4)
  line L142 (214.5, -4) -> (223, -4)
  line L143 (223, -4) -> (223, -46)
  line L144 (210.5, -46) -> (202, -46)
  line L145 (202, -46) -> (202, -4)
  line L146 (202, -4) -> (210.5, -4)
  line L147 (210.5, -4) -> (210.5, -46)
  line L148 (208.4595, -46) -> (206.25, -35.0827)
  line L149 (204.2095, -25) -> (202, -14.0827)
  line L150 (210.5, -35.9173) -> (208.2905, -25)
  line L151 (206.25, -14.9173) -> (204.0405, -4)
  line L152 (210.5, -14.0827) -> (208.2905, -25)
  line L153 (206.25, -35.0827) -> (204.0405, -46)
  line L154 (208.4595, -4) -> (206.25, -14.9173)
  line L155 (204.2095, -25) -> (202, -35.9173)
  line L156 (220.9595, -46) -> (218.75, -35.0827)
  line L157 (218.75, -35.0827) -> (216.5405, -46)
  line L158 (223, -35.9173) -> (220.7905, -25)
  line L159 (223, -14.0827) -> (220.7905, -25)
  line L160 (220.9595, -4) -> (218.75, -14.9173)
  line L161 (218.75, -14.9173) -> (216.5405, -4)
  line L162 (216.7095, -25) -> (214.5, -14.0827)
  line L163 (216.7095, -25) -> (214.5, -35.9173)
  line L164 (233.4595, -46) -> (231.25, -35.0827)
  line L165 (231.25, -35.0827) -> (229.0405, -46)
  line L166 (235.5, -35.9173) -> (233.2905, -25)
  line L167 (235.5, -14.0827) -> (233.2905, -25)
  line L168 (233.4595, -4) -> (231.25, -14.9173)
  line L169 (231.25, -14.9173) -> (229.0405, -4)
  line L170 (229.2095, -25) -> (227, -14.0827)
  line L171 (229.2095, -25) -> (227, -35.9173)
  line L172 (245.9595, -46) -> (243.75, -35.0827)
  line L173 (243.75, -35.0827) -> (241.5405, -46)
  line L174 (248, -35.9173) -> (245.7905, -25)
  line L175 (248, -14.0827) -> (245.7905, -25)
  line L176 (245.9595, -4) -> (243.75, -14.9173)
  line L177 (243.75, -14.9173) -> (241.5405, -4)
  line L178 (241.7095, -25) -> (239.5, -14.0827)
  line L179 (241.7095, -25) -> (239.5, -35.9173)
  arc A2 (248, -20.4174) -> (248, -29.5826) centre (250, -25) ccw projected
  line L180 (250, -25) -> (250, -22.497)
  arc A3 (252, -29.5826) -> (252, -20.4174) centre (250, -25) ccw
  line L181 (252, -35.9173) -> (254.2095, -25)
  line L182 (252, -14.0827) -> (254.2095, -25)
  point P0 (52, 13.6965)
  point P1 (98, 13.6965)
  point P2 (52, 6.1505)
  point P3 (123, 6.3035)
  point P4 (127, 13.6889)
  point P5 (127, 6.3035)
  point P6 (148, 13.6965)
  point P7 (102, 13.9331)
  point P8 (127, 4)
  point P9 (152, 13.2782)
  point P10 (169, 18)
  point P11 (182, 6.7218)
  point P12 (186, 13.1716)
  point P13 (198, 6.8284)
  point P14 (235.5, 7.4601)
  point P15 (227, 12.5399)
  point P16 (214.5, 12.5399)
  point P17 (223, 7.4601)
  point P18 (202, 12.5399)
  point P19 (210.5, 7.4601)
  point P20 (169, -12)
  point P21 (152, -16.7218)
  point P22 (148, -16.3035)
  point P23 (127, -26)
  point P24 (127, -23.6965)
  point P25 (127, -16.3111)
  point P26 (123, -23.6965)
  point P27 (102, -16.0669)
  point P28 (98, -16.3035)
  point P29 (52, -16.3035)
  point P30 (52, -23.8495)
  point P31 (48, -14)
  point P32 (246.5164, -28.5868)
  point P33 (246.5164, -21.4132)
  point P34 (194.08, -25)
  point P35 (192, -17.7199)
  point P36 (192, -32.2801)
  point P37 (189.92, -25)
  point P38 (137.5, -20.5279)
  point P39 (139.7361, -25)
  point P40 (137.5, -29.4721)
  point P41 (135.2639, -25)
  point P42 (112.5, -29.4721)
  point P43 (114.7361, -25)
  point P44 (110.2639, -25)
  point P45 (112.5, -20.5279)
  point P46 (87.5, -29.4721)
  point P47 (79.2361, -46)
  point P48 (89.7361, -25)
  point P49 (87.5, -20.5279)
  point P50 (79.2361, -4)
  point P51 (77, -41.5279)
  point P52 (85.2639, -25)
  point P53 (77, -8.4721)
  point P54 (77, -14)
  point P55 (77, -20)
  point P56 (77, -26)
  point P57 (64.7361, -25)
  point P58 (73, -26)
  point P59 (73, -14)
  point P60 (62.5, -20.5279)
  point P61 (70.7639, -4)
  point P62 (52, -41.5279)
  point P63 (60.2639, -25)
  point P64 (62.5, -29.4721)
  point P65 (54.2361, -46)
  point P66 (253.4836, -21.4132)
  point P67 (253.4836, -28.5868)
  dimension "d180" = 12
  dimension "d181" = 12
  dimension "d182" = 13
  dimension "d183" = 12
  dimension "d184" = 4
  dimension "d185" = 4
  dimension "d186" = 8.5
  dimension "d187" = 12
  dimension "d188" = 8.5
  dimension "d189" = 12
  dimension "d190" = 4
  dimension "d191" = 12.5
  dimension "d201" = 4
  dimension "d204" = 30
  dimension "d209" = 21
  dimension "d210" = 2
  dimension "d211" = 4
  dimension "d214" = 25
  dimension "d221" = 25
  dimension "d226" = 13
  dimension "d228" = 4
  dimension "d231" = 17
  dimension "d236" = 2
  dimension "d237" = 4
  dimension "d242" = 12.5
  constraints: 350 end point, 54 point on line, 52 parallel, 19 symmetric about line, 17 horizontal, 15 perpendicular, 8 horizontal alignment, 4 vertical, 3 midpoint, 2 point on circle, 1 centre point, 196 other
  measures "d180" distance of L11.end L12.start
  measures "d181" distance of L11.start L11.end
  measures "d182" distance of L13.end L14.start
  measures "d183" distance of L13.start L13.end
  measures "d184" distance between parallel lines of L16 L13
  measures "d185" distance between parallel lines of L11 L15
  measures "d186" distance of L18.start L17.end
  measures "d187" distance of L17.end L17.start
  measures "d188" distance of L20.start L19.end
  measures "d189" distance of L19.end L19.start
  measures "d190" distance between parallel lines of L17 L20
  measures "d191" distance of L19.start L21.start
  measures "d201" distance between parallel lines of L10 L3
  measures "d204" distance of L16.start L31.start
  measures "d210" distance between parallel lines of L91 L99
  measures "d211" distance between parallel lines of L99 L100
  measures "d214" distance of L100.start L103.start
  measures "d221" distance of L100.start L107.start
  measures "d226" distance between parallel lines of L15 L16
  measures "d228" distance between parallel lines of L119 L120
  measures "d231" distance of L119.start L126.start
  measures "d236" distance between parallel lines of L96 L132
  measures "d237" distance between parallel lines of L132 L133
  measures "d242" distance of L148.start L156.start
extrude "押し出し11" cut sketch "SCfronNNhukin" against normal through all contours L148 L220 L218 L146 | L146 L218 L148 | L158 L155 L154 | L154 L156 L155 L158 | L148 L210 L140 L145 | L145 L140 L148 | L151 L153 L161 | L148 L207 L218 L220 | L145 L138 L144 | L144 L219 L138 L145 | L136 L210 L211 L216 L144 | L145 L210 L212 L148 L140 | L140 L210 L145 | L148 L208 L140 L210 | L209 L144 L138 L145 L219 L142 | L142 L219 L209 | L141 L219 L218 L207 | L146 L211 L144 | L144 L216 L211 L146 | L144 L207 L138 L219 | L138 L219 L145 | L120 L232 L228 L231 L122 | L136 L211 L210 | L122 L121 L226 L225 | L140 L208 L145 L210 | L145 L208 L212 L210 | L197 L217 L140 L208 | L218 L219 L141 | L219 L145 L207 L142 | L142 L207 L209 L219 | L209 L220 L140 L146 | L146 L140 L195 L209 | L194 L220 L138 L207 | L138 L207 L145 L219 | L174 L286 L180 | L120 L228 L232 | L231 L228 L122 | L180 L175 L255 L177 L269 | L122 L226 L121 | L226 L121 L227 L124 L225 | L224 L226 L123 | L140 L217 L145 L208 | L145 L217 L138 L212 L208 | L197 L140 L217 | L207 L145 L220 L142 | L142 L220 L140 L209 L207 | L146 L195 L140 | L140 L220 L142 L194 L195 L146 | L209 L140 L220 | L194 L138 L220 | L138 L220 L145 L207 | L119 L301 L116 | L116 L118 L311 L115 L310 | L177 L255 L269 | L271 L176 L178 | L180 L255 L175 | L226 L122 L235 L227 L121 | L124 L227 L225 | L226 L224 L227 L125 L123 | L140 L197 L145 L217 | L145 L197 L196 L146 L138 L217 | L220 L145 L194 L142 | L212 L146 L138 L196 | L212 L217 L138 L146 | L194 L145 L220 L138 | L313 L117 L114 | L115 L311 L310 | L116 L311 L118 | L227 L235 L121 | L121 L235 L234 L124 L227 | L124 L234 L225 L227 | L224 L125 L227 | L217 L212 L138 | L138 L146 L196 | L284 L175 L251 | L229 L232 L124 L230 L121 | L121 L230 L229 | L229 L125 L124 L232 | L229 L230 L121 L241 | L262 L278 L177 | L177 L278 L176 L262 | L294 L118 L296 L116 | L300 L118 L288 | L300 L117 L115 L288 L118 | L176 L177 L251 L175 L284 | L260 L175 L276 L180 | L302 L307 L115 | L115 L307 L117 L302 | L230 L124 L241 L121 | L232 L125 L241 L230 L124 | L124 L125 L232 | L124 L230 L241 | L294 L296 L118 | L176 L251 L177 | L260 L276 L175 | L116 L305 L118 L304 | L118 L305 L115 L304 | L115 L117 L288 | L115 L305 L304 | L297 L118 L292 | L118 L297 L115 L292 | L292 L115 L297 L117
mirror "ミラー2" about plane through (0, 0, 0) normal (1, 0, 0) of "押し出し11"
extrude "押し出し12" cut sketch "SCBottom" against normal through all contours L44 L101 L100 | L99 L90 L43 L49 | L102 L99 L45 | L49 L43 L90 L101 | L102 L47 L42 L90 | L90 L42 L47 L100 | L44 L106 L103 | L104 L90 L41 L40 L53 | L90 L106 L53 L41 | L105 L104 L45 | L105 L51 L39 L90 | L90 L39 L51 L103 | L44 L114 L111 | L112 L90 L38 L57 | L90 L114 L57 L38 | L113 L112 L45 | L113 L55 L37 L36 L90 | L90 L36 L55 L111 | L44 L118 L115 | L116 L90 L35 L61 | L90 L118 L61 L35 | L117 L116 L45 | L117 L59 L34 L90 | L90 L34 L59 L115 | L44 L123 L120 | L119 L90 L33 L65 | L90 L124 L65 L33 | L122 L119 L45 | L121 L63 L32 L90 | L90 L32 L63 L120 | L44 L131 L129 | L126 L90 L31 L69 | L90 L128 L69 L31 | L127 L126 L45 | L130 L67 L90 | L90 L67 L129 | L90 L134 L73 | L73 L132 L90 | L135 L132 L45 | L44 L134 L133 | L135 L71 L90 | L90 L71 L133 | L153 L148 L45 | L97 L90 L155 | L44 L154 L151 | L149 L90 L97 | L152 L77 L90 | L90 L77 L150 | L157 L156 L45 | L75 L90 L163 | L75 L162 L90 | L44 L160 L161 | L159 L81 L90 | L90 L81 L158 | L90 L171 L79 | L79 L170 L90 | L165 L164 L45 | L44 L168 L169 | L167 L85 L90 | L90 L85 L166 | L90 L179 L83 | L83 L178 L90 | L173 L172 L45 | L44 L176 L177 | L175 L89 A0 | A0 L89 L174
extrude "押し出し13" add sketch "SCBottom" against normal blind 4 contours L90 L174 A0 | A0 L175 L90
extrude "押し出し14" add sketch "SCBottom" against normal blind 20 contours L90 L174 A0 | A0 L175 L90
extrude "押し出し15" cut sketch "SCBottom" against normal blind 16 contours L90 L174 A0 | A0 L175 L90
extrude "押し出し16" add sketch "SCBottom" against normal blind 4 contours L90 L174 A0 | A0 L175 L90
extrude "押し出し17" cut sketch "SCtop" against normal through all contours L118 L120 L114 | L117 L120 L119 | L118 L115 L121 | L121 L116 L119
mirror "ミラー3" about plane through (0, 0, 0) normal (1, 0, 0) of "押し出し12", "押し出し17"
extrude "押し出し18" add sketch "SCBottom" against normal blind 20 contours L181 L182 A1
extrude "押し出し19" cut sketch "SCBottom" against normal blind 16 contours L181 L182 A1
extrude "押し出し20" add sketch "SCBottom" against normal blind 4 contours L181 L182 A1
extrude "押し出し21" cut sketch "スケッチ7" against normal blind 2 contours A2
